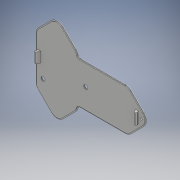
# Autodesk Inventor part: Arduino simple 4 channel ttl top Mega
Saved by Autodesk Inventor 2017 (Build 210142000, 142)
## iProperties
Created: 2016-10-04
Part Number: Arduino simple 4 channel ttl top Mega
Material: Generic
Document SubType Name: Modeling
Designer: andrew
Density: 1 g/cm^3
Appearance: Default
Author: andrew
Autodesk Inventor part; units mm, degrees
sketch "Sketch1" plane through (0, 0, 0) normal (0, 1, 0) x (-1, 0, 0)
  line L0 (70.1002, -51.1999) -> (70.1002, -37.9894) construction
  line L1 (70.1002, -37.9894) -> (68.1002, -37.9894) construction
  line L2 (68.1002, -37.9894) -> (68.1002, -48.1999) construction
  arc A0 (67.1002, -49.1999) -> (68.1002, -48.1999) centre (67.1002, -48.1999) ccw construction
  line L3 (67.1002, -49.1999) -> (-5.9213, -49.1999) construction
  arc A1 (-7.3356, -48.6141) -> (-5.9213, -49.1999) centre (-5.9213, -47.1999) ccw construction
  line L4 (-7.3356, -48.6141) -> (-7.664, -48.2857) construction
  arc A2 (-7.664, -48.2857) -> (-9.0782, -47.6999) centre (-9.0782, -49.6999) ccw construction
  line L5 (-9.0782, -47.6999) -> (-35.9958, -47.6999) construction
  arc A3 (-42.0062, -45.2103) -> (-35.9958, -47.6999) centre (-35.9958, -39.1999) ccw construction
  line L6 (-42.0062, -45.2103) -> (-62.1562, -25.0603) construction
  arc A4 (-62.1562, -13.0395) -> (-62.1562, -25.0603) centre (-56.1458, -19.0499) ccw construction
  line L7 (-62.1562, -13.0395) -> (-42.0062, 7.1105) construction
  arc A5 (-35.9958, 9.6001) -> (-42.0062, 7.1105) centre (-35.9958, 1.1001) ccw construction
  line L8 (-35.9958, 9.6001) -> (-9.0782, 9.6001) construction
  arc A6 (-9.0782, 9.6001) -> (-7.664, 10.1859) centre (-9.0782, 11.6001) ccw construction
  line L9 (-7.664, 10.1859) -> (-7.3356, 10.5143) construction
  arc A7 (-5.9213, 11.1001) -> (-7.3356, 10.5143) centre (-5.9213, 9.1001) ccw construction
  line L10 (-5.9213, 11.1001) -> (67.1002, 11.1001) construction
  arc A8 (68.1002, 10.1001) -> (67.1002, 11.1001) centre (67.1002, 10.1001) ccw construction
  line L11 (68.1002, 10.1001) -> (68.1002, 5.7045) construction
  line L12 (68.1002, 5.7045) -> (70.1002, 5.7045) construction
  line L13 (70.1002, 5.7045) -> (70.1002, 13.1001) construction
  line L14 (70.1002, 13.1001) -> (-35.9958, 13.1001) construction
  arc A9 (-35.9958, 13.1001) -> (-44.4811, 9.5854) centre (-35.9958, 1.1001) ccw construction
  line L15 (-44.4811, 9.5854) -> (-64.6311, -10.5646) construction
  arc A10 (-64.6311, -10.5646) -> (-64.6311, -27.5352) centre (-56.1458, -19.0499) ccw construction
  line L16 (-64.6311, -27.5352) -> (-44.4811, -47.6852) construction
  arc A11 (-44.4811, -47.6852) -> (-35.9958, -51.1999) centre (-35.9958, -39.1999) ccw construction
  line L17 (-35.9958, -51.1999) -> (70.1002, -51.1999) construction
  line L18 (70.1002, -21.9894) -> (70.1002, -6.0043) construction
  line L19 (70.1002, -6.0043) -> (68.1002, -6.0043) construction
  line L20 (68.1002, -6.0043) -> (68.1002, -21.9894) construction
  line L21 (68.1002, -21.9894) -> (70.1002, -21.9894) construction
  line L22 (71.1002, -21.9894) -> (71.1002, -6.0043) construction
  line L23 (71.1002, 5.7045) -> (71.1002, 13.1001)
  arc A12 (71.1002, 13.1001) -> (70.1002, 14.1001) centre (70.1002, 13.1001) ccw construction
  line L24 (70.1002, 14.1001) -> (-35.9958, 14.1001) construction
  arc A13 (-35.9958, 14.1001) -> (-45.1882, 10.2925) centre (-35.9958, 1.1001) ccw construction
  line L25 (-45.1882, 10.2925) -> (-65.3382, -9.8575) construction
  arc A14 (-65.3382, -9.8575) -> (-65.3382, -28.2423) centre (-56.1458, -19.0499) ccw construction
  line L26 (-65.3382, -28.2423) -> (-45.1882, -48.3923) construction
  arc A15 (-45.1882, -48.3923) -> (-35.9958, -52.1999) centre (-35.9958, -39.1999) ccw construction
  line L27 (-35.9958, -52.1999) -> (70.1002, -52.1999) construction
  arc A16 (70.1002, -52.1999) -> (71.1002, -51.1999) centre (70.1002, -51.1999) ccw construction
  line L28 (71.1002, -51.1999) -> (71.1002, -37.9894)
  line L29 (71.1002, -37.9894) -> (70.1002, -37.9894) construction
  line L30 (70.1002, -37.9894) -> (70.1002, -51.1999) construction
  line L31 (70.1002, -51.1999) -> (-35.9958, -51.1999) construction
  arc A17 (-44.4811, -47.6852) -> (-35.9958, -51.1999) centre (-35.9958, -39.1999) ccw construction
  line L32 (-44.4811, -47.6852) -> (-64.6311, -27.5352) construction
  arc A18 (-64.6311, -10.5646) -> (-64.6311, -27.5352) centre (-56.1458, -19.0499) ccw construction
  line L33 (-64.6311, -10.5646) -> (-44.4811, 9.5854) construction
  arc A19 (-35.9958, 13.1001) -> (-44.4811, 9.5854) centre (-35.9958, 1.1001) ccw construction
  line L34 (-35.9958, 13.1001) -> (70.1002, 13.1001) construction
  line L35 (70.1002, 13.1001) -> (70.1002, 5.7045) construction
  line L36 (70.1002, 5.7045) -> (71.1002, 5.7045) construction
  line L37 (71.1002, 5.7045) -> (71.1002, 13.1001) construction
  line L38 (71.1002, 5.7045) -> (71.1002, -37.9894)
  arc A20 (-62.1562, -13.0395) -> (-62.1562, -25.0603) centre (-56.1458, -19.0499) ccw construction
  line L39 (-64.6458, -19.0499) -> (-76.6779, -19.0499) construction
  arc A21 (-65.3382, -9.8575) -> (-65.3382, -28.2423) centre (-56.1458, -19.0499) ccw construction
  circle A22 centre (-63.0458, -19.0499) radius 1.8 construction
  circle A23 centre (-95.1541, -19.0499) radius 1.6
  line L40 (-91.8832, -9.7665) -> (-75.0062, 7.1105) construction
  arc A24 (-68.9958, 9.6001) -> (-75.0062, 7.1105) centre (-68.9958, 1.1001) ccw construction
  line L41 (-68.9958, 9.6001) -> (-42.4924, 9.6001) construction
  arc A25 (-42.4924, 9.6001) -> (-40.3711, 10.4788) centre (-42.4924, 12.6001) ccw construction
  line L42 (-40.3711, 10.4788) -> (-40.6284, 10.2214) construction
  arc A26 (-38.5071, 11.1001) -> (-40.6284, 10.2214) centre (-38.5071, 8.1001) ccw construction
  line L43 (-38.5071, 11.1001) -> (6.3002, 11.1001) construction
  arc A27 (6.3002, 11.1001) -> (9.3002, 14.1001) centre (6.3002, 14.1001) ccw construction
  arc A28 (11.7898, 20.1105) -> (9.3002, 14.1001) centre (17.8002, 14.1001) ccw construction
  line L44 (11.7898, 20.1105) -> (31.9398, 40.2605) construction
  arc A29 (43.9606, 40.2605) -> (31.9398, 40.2605) centre (37.9502, 34.2501) ccw construction
  line L45 (43.9606, 40.2605) -> (64.1106, 20.1105) construction
  arc A30 (66.5817, 14.6605) -> (64.1106, 20.1105) centre (58.1002, 14.1001) ccw construction
  line L46 (66.5817, 14.6605) -> (68.1002, 10.3919) construction
  line L47 (68.1002, 10.3919) -> (68.1002, 5.7045) construction
  line L48 (68.1002, 5.7045) -> (70.1002, 5.7045) construction
  line L49 (70.1002, 5.7045) -> (70.1002, 14.1001) construction
  arc A31 (70.1002, 14.1001) -> (66.5855, 22.5854) centre (58.1002, 14.1001) ccw construction
  line L50 (66.5855, 22.5854) -> (46.4355, 42.7354) construction
  arc A32 (46.4355, 42.7354) -> (29.4649, 42.7354) centre (37.9502, 34.2501) ccw construction
  line L51 (29.4649, 42.7354) -> (9.3149, 22.5854) construction
  arc A33 (9.3149, 22.5854) -> (6.0131, 16.3501) centre (17.8002, 14.1001) ccw construction
  arc A34 (2.084, 13.1001) -> (6.0131, 16.3501) centre (2.084, 17.1001) ccw construction
  line L52 (2.084, 13.1001) -> (-68.9958, 13.1001) construction
  arc A35 (-68.9958, 13.1001) -> (-77.4811, 9.5854) centre (-68.9958, 1.1001) ccw construction
  line L53 (-77.4811, 9.5854) -> (-97.6311, -10.5646) construction
  arc A36 (-97.6311, -10.5646) -> (-97.6311, -27.5352) centre (-89.1458, -19.0499) ccw construction
  line L54 (-97.6311, -27.5352) -> (-77.481, -47.6852) construction
  arc A37 (-77.481, -47.6852) -> (-68.9958, -51.1999) centre (-68.9958, -39.1999) ccw construction
  line L55 (-68.9958, -51.1999) -> (2.084, -51.1999) construction
  arc A38 (6.0131, -54.4499) -> (2.084, -51.1999) centre (2.084, -55.1999) ccw construction
  arc A39 (6.0131, -54.4499) -> (9.3149, -60.6852) centre (17.8002, -52.1999) ccw construction
  line L56 (9.3149, -60.6852) -> (29.4649, -80.8352) construction
  arc A40 (29.4649, -80.8352) -> (46.4355, -80.8352) centre (37.9502, -72.3499) ccw construction
  line L57 (46.4355, -80.8352) -> (66.5855, -60.6852) construction
  arc A41 (66.5855, -60.6852) -> (70.1002, -52.1999) centre (58.1002, -52.1999) ccw construction
  line L58 (70.1002, -52.1999) -> (70.1002, -37.9894) construction
  line L59 (70.1002, -37.9894) -> (68.1002, -37.9894) construction
  line L60 (68.1002, -37.9894) -> (68.1002, -49.1999) construction
  line L61 (68.1002, -49.1999) -> (66.8919, -51.6165) construction
  arc A42 (64.1106, -58.2103) -> (66.8919, -51.6165) centre (57.0713, -51.3576) ccw construction
  line L62 (64.1106, -58.2103) -> (43.9606, -78.3603) construction
  arc A43 (31.9398, -78.3603) -> (43.9606, -78.3603) centre (37.9502, -72.3499) ccw construction
  line L63 (31.9398, -78.3603) -> (11.7898, -58.2103) construction
  arc A44 (9.3002, -52.1999) -> (11.7898, -58.2103) centre (17.8002, -52.1999) ccw construction
  arc A45 (9.3002, -52.1999) -> (6.3002, -49.1999) centre (6.3002, -52.1999) ccw construction
  line L64 (6.3002, -49.1999) -> (-38.9213, -49.1999) construction
  arc A46 (-40.3356, -48.6141) -> (-38.9213, -49.1999) centre (-38.9213, -47.1999) ccw construction
  line L65 (-40.3356, -48.6141) -> (-40.3711, -48.5786) construction
  arc A47 (-40.3711, -48.5786) -> (-42.4924, -47.6999) centre (-42.4924, -50.6999) ccw construction
  line L66 (-42.4924, -47.6999) -> (-68.9958, -47.6999) construction
  arc A48 (-75.0062, -45.2103) -> (-68.9958, -47.6999) centre (-68.9958, -39.1999) ccw construction
  line L67 (-75.0062, -45.2103) -> (-91.4374, -28.7791) construction
  line L68 (-91.4374, -28.7791) -> (-91.4374, -10.2123) construction
  line L69 (-91.4374, -10.2123) -> (-91.8832, -9.7665) construction
  arc A49 (-68.9958, 14.1001) -> (-78.1882, 10.2925) centre (-68.9958, 1.1001) ccw
  line L70 (-78.1882, 10.2925) -> (-98.3382, -9.8575)
  arc A50 (-98.3382, -9.8575) -> (-98.3382, -28.2423) centre (-89.1458, -19.0499) ccw
  line L71 (-98.3382, -28.2423) -> (-78.1882, -48.3923)
  arc A51 (-78.1882, -48.3923) -> (-68.9958, -52.1999) centre (-68.9958, -39.1999) ccw
  line L72 (-68.9958, -52.1999) -> (2.084, -52.1999)
  arc A52 (5.0308, -54.6374) -> (2.084, -52.1999) centre (2.084, -55.1999) ccw
  arc A53 (5.0308, -54.6374) -> (8.6078, -61.3923) centre (17.8002, -52.1999) ccw
  line L73 (8.6078, -61.3923) -> (28.7578, -81.5423)
  arc A54 (28.7578, -81.5423) -> (47.1426, -81.5423) centre (37.9502, -72.3499) ccw
  line L74 (47.1426, -81.5423) -> (67.2926, -61.3923)
  arc A55 (67.2926, -61.3923) -> (71.1002, -52.1999) centre (58.1002, -52.1999) ccw
  line L75 (71.1002, -52.1999) -> (71.1002, -37.9894)
  line L76 (71.1002, -37.9894) -> (70.1002, -37.9894) construction
  line L77 (70.1002, -37.9894) -> (70.1002, -52.1999) construction
  arc A56 (66.5855, -60.6852) -> (70.1002, -52.1999) centre (58.1002, -52.1999) ccw construction
  line L78 (66.5855, -60.6852) -> (46.4355, -80.8352) construction
  arc A57 (29.4649, -80.8352) -> (46.4355, -80.8352) centre (37.9502, -72.3499) ccw construction
  line L79 (29.4649, -80.8352) -> (9.3149, -60.6852) construction
  arc A58 (6.0131, -54.4499) -> (9.3149, -60.6852) centre (17.8002, -52.1999) ccw construction
  arc A59 (6.0131, -54.4499) -> (2.084, -51.1999) centre (2.084, -55.1999) ccw construction
  line L80 (2.084, -51.1999) -> (-68.9958, -51.1999) construction
  arc A60 (-77.481, -47.6852) -> (-68.9958, -51.1999) centre (-68.9958, -39.1999) ccw construction
  line L81 (-77.481, -47.6852) -> (-97.6311, -27.5352) construction
  arc A61 (-97.6311, -10.5646) -> (-97.6311, -27.5352) centre (-89.1458, -19.0499) ccw construction
  line L82 (-97.6311, -10.5646) -> (-77.4811, 9.5854) construction
  arc A62 (-68.9958, 13.1001) -> (-77.4811, 9.5854) centre (-68.9958, 1.1001) ccw construction
  line L83 (-68.9958, 13.1001) -> (2.084, 13.1001) construction
  arc A63 (2.084, 13.1001) -> (6.0131, 16.3501) centre (2.084, 17.1001) ccw construction
  arc A64 (9.3149, 22.5854) -> (6.0131, 16.3501) centre (17.8002, 14.1001) ccw construction
  line L84 (9.3149, 22.5854) -> (29.4649, 42.7354) construction
  arc A65 (46.4355, 42.7354) -> (29.4649, 42.7354) centre (37.9502, 34.2501) ccw construction
  line L85 (46.4355, 42.7354) -> (66.5855, 22.5854) construction
  arc A66 (70.1002, 14.1001) -> (66.5855, 22.5854) centre (58.1002, 14.1001) ccw construction
  line L86 (70.1002, 14.1001) -> (70.1002, 5.7045) construction
  line L87 (70.1002, 5.7045) -> (71.1002, 5.7045) construction
  line L88 (71.1002, 5.7045) -> (71.1002, 14.1001)
  arc A67 (71.1002, 14.1001) -> (67.2926, 23.2925) centre (58.1002, 14.1001) ccw
  line L89 (67.2926, 23.2925) -> (47.1426, 43.4425)
  arc A68 (47.1426, 43.4425) -> (28.7578, 43.4425) centre (37.9502, 34.2501) ccw
  line L90 (28.7578, 43.4425) -> (8.6078, 23.2925)
  arc A69 (8.6078, 23.2925) -> (5.0308, 16.5376) centre (17.8002, 14.1001) ccw
  arc A70 (2.084, 14.1001) -> (5.0308, 16.5376) centre (2.084, 17.1001) ccw
  line L91 (2.084, 14.1001) -> (-68.9958, 14.1001)
  line L92 (70.1002, -21.9894) -> (70.1002, -6.0043) construction
  line L93 (70.1002, -6.0043) -> (68.1002, -6.0043) construction
  line L94 (68.1002, -6.0043) -> (68.1002, -21.9894) construction
  line L95 (68.1002, -21.9894) -> (70.1002, -21.9894) construction
  line L96 (70.1002, -6.0043) -> (70.1002, -21.9894) construction
  line L97 (70.1002, -21.9894) -> (71.1002, -21.9894) construction
  line L98 (71.1002, -21.9894) -> (71.1002, -6.0043) construction
  line L99 (71.1002, -6.0043) -> (70.1002, -6.0043) construction
  point P0 (0, 0)
  point P1 (66.1, 7.6)
  point P2 (-59.329, -19.0499)
  point P3 (66.1, 7.6)
  constraints: 200 end point, 139 point on circle, 71 centre point, 1 coincident, 1 vertical
extrude "Extrusion1" add sketch "Sketch1" along normal blind 3
sketch "Sketch2" plane through (0, 0, 0) normal (0, -1, 0) x (1, 0, 0)
  circle A0 centre (95.1541, -19.0499) radius 1.6 projected
  arc A1 (-67.2926, 23.2925) -> (-71.1002, 14.1001) centre (-58.1002, 14.1001) ccw projected
  line L0 (-71.1002, 14.1001) -> (-71.1002, -52.1999) projected
  arc A2 (-71.1002, -52.1999) -> (-67.2926, -61.3923) centre (-58.1002, -52.1999) ccw projected
  line L1 (-67.2926, -61.3923) -> (-47.1426, -81.5423) projected
  arc A3 (-47.1426, -81.5423) -> (-28.7578, -81.5423) centre (-37.9502, -72.3499) ccw projected
  line L2 (-28.7578, -81.5423) -> (-8.6078, -61.3923) projected
  arc A4 (-8.6078, -61.3923) -> (-5.0308, -54.6374) centre (-17.8002, -52.1999) ccw projected
  arc A5 (-2.084, -52.1999) -> (-5.0308, -54.6374) centre (-2.084, -55.1999) ccw projected
  line L3 (-2.084, -52.1999) -> (68.9958, -52.1999) projected
  arc A6 (68.9958, -52.1999) -> (78.1882, -48.3923) centre (68.9958, -39.1999) ccw projected
  line L4 (78.1882, -48.3923) -> (98.3382, -28.2423) projected
  arc A7 (98.3382, -28.2423) -> (98.3382, -9.8575) centre (89.1458, -19.0499) ccw projected
  line L5 (98.3382, -9.8575) -> (78.1882, 10.2925) projected
  arc A8 (78.1882, 10.2925) -> (68.9958, 14.1001) centre (68.9958, 1.1001) ccw projected
  line L6 (68.9958, 14.1001) -> (-2.084, 14.1001) projected
  arc A9 (-5.0308, 16.5376) -> (-2.084, 14.1001) centre (-2.084, 17.1001) ccw projected
  arc A10 (-5.0308, 16.5376) -> (-8.6078, 23.2925) centre (-17.8002, 14.1001) ccw projected
  line L7 (-8.6078, 23.2925) -> (-28.7578, 43.4425) projected
  arc A11 (-28.7578, 43.4425) -> (-47.1426, 43.4425) centre (-37.9502, 34.2501) ccw projected
  line L8 (-47.1426, 43.4425) -> (-67.2926, 23.2925) projected
  line L9 (-46.082, -80.4816) -> (-66.232, -60.3316)
  arc A12 (-69.6002, -52.1999) -> (-66.232, -60.3316) centre (-58.1002, -52.1999) ccw
  line L10 (-69.6002, -52.1999) -> (-69.6002, 14.1001)
  arc A13 (-66.232, 22.2318) -> (-69.6002, 14.1001) centre (-58.1002, 14.1001) ccw
  line L11 (-66.232, 22.2318) -> (-46.082, 42.3818)
  arc A14 (-29.8185, 42.3818) -> (-46.082, 42.3818) centre (-37.9502, 34.2501) ccw
  line L12 (-29.8185, 42.3818) -> (-9.6685, 22.2318)
  arc A15 (-6.5042, 16.2563) -> (-9.6685, 22.2318) centre (-17.8002, 14.1001) ccw
  arc A16 (-6.5042, 16.2563) -> (-2.084, 12.6001) centre (-2.084, 17.1001) ccw
  line L13 (-2.084, 12.6001) -> (68.9958, 12.6001)
  arc A17 (77.1275, 9.2318) -> (68.9958, 12.6001) centre (68.9958, 1.1001) ccw
  line L14 (77.1275, 9.2318) -> (97.2775, -10.9182)
  arc A18 (97.2775, -27.1816) -> (97.2775, -10.9182) centre (89.1458, -19.0499) ccw
  line L15 (97.2775, -27.1816) -> (77.1275, -47.3316)
  arc A19 (68.9958, -50.6999) -> (77.1275, -47.3316) centre (68.9958, -39.1999) ccw
  line L16 (68.9958, -50.6999) -> (-2.084, -50.6999)
  arc A20 (-2.084, -50.6999) -> (-6.5042, -54.3562) centre (-2.084, -55.1999) ccw
  arc A21 (-9.6685, -60.3316) -> (-6.5042, -54.3562) centre (-17.8002, -52.1999) ccw
  line L17 (-9.6685, -60.3316) -> (-29.8185, -80.4816)
  arc A22 (-46.082, -80.4816) -> (-29.8185, -80.4816) centre (-37.9502, -72.3499) ccw
  dimension "d73" = 1.5
  constraints: 22 point on circle, 18 end point, 11 centre point, 19 other
  measures "d73" distance between parallel lines of L1 L9
extrude "Extrusion2" cut sketch "Sketch2" against normal blind 1 contours L8 A11 L7 A10 A9 L6 A8 L5 A7 L4 A6 L3 A5 A4 L2 A3 L1 A2 L0 A1
fillet "Fillet1" radius 2 3 edges at (33.4559, 3, -52.1999) (-71.1002, 3, -19.0499) (33.4559, 3, 14.1001)
ref_plane "Work Plane2" through (-66.7002, 0, -21.9095) normal (0, 0, -1) x (-1, 0, 0)
ref_plane "Work Plane3" through (-66.7002, 0, -21.9095) normal (0, 0, -1) x (-1, 0, 0)
ref_plane "Work Plane1" through (58.929, 0, -27.4875) normal (0, 0, -1) x (-1, 0, 0)
ref_plane "Work Plane5" through (58.929, 0, -27.4875) normal (0, 0, -1) x (-1, 0, 0)
sketch "Sketch10" plane through (58.929, 0, -27.4875) normal (0, 0, -1) x (-1, 0, 0)
  line L0 (0, -4.4643) -> (-0.9, -3.5) projected
  line L1 (-0.45, -3.9821) -> (1.0587, -5.5986)
  line L2 (1.0587, -5.5986) -> (-0.45, -5.5986)
  line L3 (-0.45, -5.5986) -> (-0.45, -3.9821)
  point P0 (58.929, 0)
  constraints: 6 end point, 1 collinear, 1 horizontal, 1 midpoint, 1 perpendicular
extrude "Extrusion10" cut sketch "Sketch10" against normal blind 20
sketch "Sketch11" plane through (0, 3, 0) normal (0, 1, 0) x (1, 0, 0)
  arc A0 (65.3382, 9.8575) -> (65.3382, 28.2423) centre (56.1458, 19.0499) ccw construction
  arc A1 (65.3382, 9.8575) -> (65.3382, 28.2423) centre (56.1458, 19.0499) ccw construction
  circle A2 centre (-50.8, 43.1) radius 1.6 construction
  line L0 (-50.8, 43.1) -> (-59.26, 43.1) construction
  line L1 (-59.26, 43.1) -> (-59.26, 41.7) construction
  circle A3 centre (-59.26, 41.7) radius 3.25
  circle A4 centre (15.3, -50.7) radius 1.6
  circle A5 centre (14, -2.5) radius 1.6
  circle A6 centre (14, -2.5) radius 2.345
  line L2 (0, -53.3) -> (0, 0) construction
  line L3 (-1.8, -3.3) -> (0, -3.3) construction
  line L4 (-1.8, -12.2) -> (-1.8, -3.3) construction
  line L5 (0, -12.2) -> (-1.8, -12.2) construction
  line L6 (0, -43.5895) -> (0, -31.5895) construction
  line L7 (-6.2, -31.5895) -> (0, -31.5895) construction
  line L8 (0, -43.5895) -> (-6.2, -43.5895) construction
  line L9 (-6.2, -43.5895) -> (-6.2, -31.5895) construction
  line L10 (-6.2, -43.5895) -> (-6.2, -31.5895) construction
  line L11 (0, -12.2) -> (0, -3.3) construction
  circle A7 centre (66.1, -35.5) radius 2.345
  circle A8 centre (15.3, -50.7) radius 2.345
  line L12 (66.1, -53.3) -> (0, -53.3) construction
  line L13 (0, 0) -> (68.6, 0) construction
  line L14 (66.1, -40.6) -> (66.1, -53.3) construction
  circle A9 centre (66.1, -35.5) radius 1.6
  circle A10 centre (66.1, -7.6) radius 1.6
  circle A11 centre (66.1, -7.6) radius 2.345
  line L15 (68.6, 0) -> (68.6, -40.6) construction
  line L16 (68.6, -40.6) -> (66.1, -40.6) construction
  line L17 (66.1, -35.5) -> (90.2, -35.5) construction
  line L18 (14, -2.5) -> (-6.2, -2.5) construction
  line L19 (0, -2.5) -> (96.52, -2.5) construction
  line L20 (0, -2.5) -> (96.52, -2.5) construction
  line L21 (90.2, -35.5) -> (90.2, -50.7) construction
  circle A12 centre (90.2, -50.7) radius 1.6
  circle A13 centre (90.2, -50.7) radius 2.345
  circle A14 centre (96.52, -2.5) radius 1.6
  circle A15 centre (96.52, -2.5) radius 2.345
  line L22 (68.6, -20.3) -> (101.6, -20.3) construction
  line L23 (101.6, -20.3) -> (101.6, 10.1637) construction
  line L24 (-71.1002, 52.1999) -> (-71.1002, -14.1001) projected
  line L25 (-71.1002, 19.0499) -> (8.0198, 19.0499) construction
  line L26 (-71.1002, 19.0499) -> (8.0198, 19.0499) construction
  circle A16 centre (8.0198, 19.0499) radius 3.25
  dimension "d42" = 8.46
  dimension "d43" = 1.4
  dimension "d44" = 6.5
  dimension "d81" = 14
  dimension "d82" = 66.1
  dimension "d83" = 2.5
  dimension "d84" = 7.6
  dimension "d85" = 35.5
  dimension "d86" = 50.7
  dimension "d87" = 24.1
  dimension "d88" = 96.52
  dimension "d89" = 0
  dimension "d90" = 15.2
  dimension "d91" = 33
  dimension "d92" = 79.12
  dimension "d93" = 0
  dimension "d94" = 6.5
  constraints: 52 end point, 16 centre point, 7 horizontal, 3 collinear, 2 coincident, 2 midpoint, 2 point on circle, 2 point on line, 2 vertical, 1 perpendicular
  measures "d42" distance of L0.start L0.end
  measures "d43" distance of L0.end L1.end
  measures "d44" diameter of A3
  measures "d81" distance from line of L2 L18.start
  measures "d82" distance from line of A10.centre L2
  measures "d83" distance from line of L13 A6.centre
  measures "d84" distance from line of L13 A10.centre
  measures "d85" distance from line of L13 A7.centre
  measures "d86" distance from line of L13 A4.centre
  measures "d87" distance of L17.start L17.end
  measures "d88" distance of L19.start L19.end
  measures "d89" distance between parallel lines of L19 L20
  measures "d90" distance of L17.end L21.end
  measures "d91" distance of L22.start L22.end
  measures "d92" distance of L25.start L25.end
  measures "d93" distance between parallel lines of L25 L26
  measures "d94" diameter of A16
extrude "Extrusion11" cut sketch "Sketch11" against normal blind 10 contours A3 | A16
chamfer "Chamfer1" distance 2 angle 45 2 edges at (-62.51, 3, -41.7) (4.7698, 3, -19.0499)
ref_plane "Work Plane4" through (-67.7002, -4.4643, -6.1514) normal (0, 0, 1) x (1, 0, 0)
sketch "Sketch13" plane through (-67.7002, -4.4643, -6.1514) normal (0, 0, 1) x (1, 0, 0)
  line L0 (0.5, -0.5357) -> (-0.9, 0.9643) construction
  line L1 (0.5, -0.5357) -> (-0.9, 0.9643) construction
  line L2 (-0.9, 1.4643) -> (-0.9, 0.9643) construction
  line L3 (-0.9, 0.9643) -> (-0.9, 1.4643) construction
  line L4 (-0.9, 1.4643) -> (0, 1.4643) construction
  line L5 (0, 4.4643) -> (3, 4.4643) construction
  line L6 (1, -0.5357) -> (2, -0.5357) construction
  line L7 (2, -0.5357) -> (4.7832, 4.4643) construction
  line L8 (3, 4.4643) -> (4.7832, 4.4643) construction
  line L9 (0, 1.4643) -> (0, 4.4643) construction
  line L10 (0, 4.4643) -> (3, 4.4643) projected
  line L11 (0, 4.4643) -> (4.7832, 4.4643)
  line L12 (1.4683, 4.4643) -> (21.6183, 4.4643) projected
  line L13 (4.7832, 4.4643) -> (2, -0.5357)
  line L14 (2, -0.5357) -> (0.5, -0.5357)
  line L15 (-0.9, 0.9643) -> (0.5, -0.5357)
  line L16 (-0.9, 0.9643) -> (-0.9, 1.4643)
  line L17 (0, 1.4643) -> (-0.9, 1.4643) projected
  line L18 (-0.9, 1.4643) -> (0, 1.4643)
  line L19 (0, 4.4643) -> (0, 0) projected
  line L20 (0, 1.4643) -> (0, 4.4643)
  point P0 (67.7002, 4.4643)
  constraints: 30 end point, 3 perpendicular, 2 horizontal, 2 parallel, 1 collinear, 1 vertical
extrude "Extrusion13" add sketch "Sketch13" against normal blind 15.758
ref_plane "Work Plane6" through (58.929, 0, -10.6125) normal (0, 0, 1) x (1, 0, 0)
sketch "Sketch14" plane through (58.929, 0, -10.6125) normal (0, 0, 1) x (1, 0, 0)
  line L0 (-124.6293, -5) -> (-126.1293, -5) projected
  line L1 (-121.8461, 0) -> (-124.6293, -5)
  line L2 (-124.6293, -5) -> (-126.1293, -5)
  line L3 (-127.5293, -3.5) -> (-127.5293, -3) projected
  line L4 (-126.1293, -5) -> (-127.5293, -3.5)
  line L5 (-127.5293, -3.5) -> (-127.5293, -3)
  line L6 (-127.5293, -3) -> (-126.6293, -3)
  line L7 (-126.6293, 0) -> (-121.8461, 0)
  line L8 (-125.161, 0) -> (-105.011, 0) projected
  line L9 (-126.6293, -3) -> (-126.6293, 0) projected
  line L10 (-126.6293, 0) -> (-126.6293, -3)
  line L11 (27.3256, 0) -> (30.1087, -5)
  line L12 (30.1087, -5) -> (31.6087, -5)
  line L13 (31.6087, -5) -> (33.0087, -3.5)
  line L14 (33.0087, -3.5) -> (33.0087, -3)
  line L15 (33.0087, -3) -> (32.1087, -3)
  line L16 (32.1087, 0) -> (27.3256, 0)
  line L17 (32.1087, 0) -> (32.1087, -3)
  line L18 (-0.5, -5) -> (0.9, -3.5) projected
  line L19 (-126.2216, 1) -> (-130.0293, 1) projected
  line L20 (-130.0293, 1) -> (-130.0293, -6.3994)
  line L21 (43.2167, 1) -> (39.4091, 1) projected
  line L22 (43.2167, 1) -> (32.1087, 1)
  line L23 (32.1087, 1) -> (32.1087, 0)
  line L24 (38.3485, 0) -> (18.1985, 0) projected
  point P0 (-58.929, 0)
  dimension "d78" = 3.4
  dimension "d79" = 11.108
  dimension "d80" = 90
  constraints: 34 end point, 5 collinear, 1 perpendicular, 1 point on line, 1 vertical
  measures "d78" distance between parallel lines of L20 L9
  measures "d79" distance of L21.start L22.end
  measures "d80" angle of L23 L22
extrude "Extrusion14" add sketch "Sketch14" against normal blind 16.875 contours L16 L17 L15 L14 L13 L12 L11
body "Solid1"
